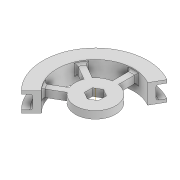
# Autodesk Inventor part: Primary_hinge_guide_pulley_fix
Saved by Autodesk Inventor 2022 (Build 260153000, 153)
## iProperties
Created: 2022-09-24
Part Number: Primary_hinge_guide_pulley_fix
Material: Generic
Document SubType Name: Modeling
Designer: dell
Density: 1 g/cm^3
Appearance: Default
Author: dell
Autodesk Inventor part; units mm, degrees
ref_plane "YZ Plane" through (0, 0, 0) normal (1, 0, 0) x (0, 1, 0)
ref_plane "XZ Plane" through (0, 0, 0) normal (0, 1, 0) x (-1, 0, 0)
ref_plane "XY Plane" through (0, 0, 0) normal (0, 0, 1) x (1, 0, 0)
sketch "Sketch1" plane through (0, 0, 0) normal (0, 1, 0) x (-1, 0, 0)
  circle A0 centre (0, 0) radius 2.05
  circle A1 centre (0, 0) radius 22
  dimension "d0" = 4.1
  dimension "d1" = 44
  constraints: 2 centre point, 2 coincident
  measures "d0" diameter of A0
  measures "d1" diameter of A1
extrude "Extrusion1" add sketch "Sketch1" along normal blind 3.7
sketch "Sketch5" plane through (0, 3.7, 0) normal (0, 1, 0) x (1, 0, 0)
  circle A0 centre (0, 0) radius 22 projected
  circle A1 centre (0, 0) radius 2.05 projected
  circle A2 centre (0, 0) radius 26
  circle A3 centre (0, 0) radius 19
  dimension "d11" = 4
  dimension "d17" = 3
  constraints: 2 centre point
  measures "d11" radial gap between concentric circles of A0 A2
  measures "d17" radial gap between concentric circles of A0 A3
extrude "Extrusion4" add sketch "Sketch5" along normal blind 1.5 contours A0 | A2
sketch "Sketch11" plane through (0, 0, 0) normal (0, -1, 0) x (1, 0, 0)
  circle A0 centre (0, 0) radius 22 projected
  circle A1 centre (0, 0) radius 2.05 projected
  circle A2 centre (0, 0) radius 19
  dimension "d38" = 3
  constraints: 1 centre point
  measures "d38" radial gap between concentric circles of A0 A2
extrude "Extrusion10" add sketch "Sketch11" along normal blind 3 contours A0
sketch "Sketch6" plane through (0, -3, 0) normal (0, -1, 0) x (1, 0, 0)
  circle A0 centre (0, 0) radius 2.05 projected
  circle A1 centre (0, 0) radius 26
  circle A2 centre (0, 0) radius 19
  constraints: 2 centre point
extrude "Extrusion5" add sketch "Sketch6" along normal blind 1.5 contours A1
sketch "Sketch7" plane through (0, 3.7, 0) normal (0, 1, 0) x (1, 0, 0)
  circle A0 centre (0, 0) radius 19
  circle A1 centre (0, 0) radius 22
  circle A2 centre (0, 0) radius 10
  line L0 (-1.5, 9.88686) -> (-1.5, 18.940697)
  circle A3 centre (0, 0) radius 19
  line L1 (1.5, 9.88686) -> (1.5, 18.940697)
  line L2 (-7.812272, 6.242468) -> (-15.653125, 10.769387)
  line L3 (-9.312272, 3.644392) -> (-17.153125, 8.17131)
  line L4 (-9.312272, -3.644392) -> (-17.153125, -8.17131)
  line L5 (-7.812272, -6.242468) -> (-15.653125, -10.769387)
  line L6 (-1.5, -9.88686) -> (-1.5, -18.940697)
  line L7 (1.5, -9.88686) -> (1.5, -18.940697)
  line L8 (7.812272, -6.242468) -> (15.653125, -10.769387)
  line L9 (9.312272, -3.644392) -> (17.153125, -8.17131)
  line L10 (9.312272, 3.644392) -> (17.153125, 8.17131)
  line L11 (7.812272, 6.242468) -> (15.653125, 10.769387)
  point P0 (1.5, 18.940697)
  point P1 (-1.5, 18.940697)
  point P2 (-9.312272, -3.644392)
  point P3 (-9.312272, 3.644392)
  point P4 (-1.5, -18.940697)
  point P5 (-1.5, -9.88686)
  point P6 (-7.812272, -6.242468)
  point P7 (-15.653125, -10.769387)
  point P8 (7.812272, -6.242468)
  point P9 (1.5, -18.940697)
  point P10 (9.312272, 3.644392)
  point P11 (7.812272, 6.242468)
  dimension "d19" = 20
  dimension "d20" = 3
  dimension "d21" = 1.5
  dimension "d26" = 360
  constraints: 24 end point, 4 point on circle, 1 centre point, 1 coincident, 1 parallel, 1 vertical, 37 other
  measures "d19" diameter of A2
  measures "d20" distance between parallel lines of L0 L1
  measures "d21" distance from line of point (0, 0) L0
extrude "Extrusion7" cut sketch "Sketch7" against normal blind 10 contours A0 L9 A2 L10 | L11 A2 L1 A0 | A0 L7 A2 L8 | L0 A2 L2 A0 | A0 L5 A2 L6 | L3 A2 L4 A0
sketch "Sketch8" plane through (0, 3.7, 0) normal (0, 1, 0) x (1, 0, 0)
  line L0 (0, -4.041452) -> (-3.5, -2.020726)
  line L1 (-3.5, -2.020726) -> (-3.5, 2.020726)
  line L2 (-3.5, 2.020726) -> (0, 4.041452)
  line L3 (0, 4.041452) -> (3.5, 2.020726)
  line L4 (3.5, 2.020726) -> (3.5, -2.020726)
  line L5 (3.5, -2.020726) -> (0, -4.041452)
  point P0 (0, 0)
  point P1 (0, 0)
  dimension "d30" = 7
  constraints: 12 end point, 1 coincident, 13 other
  measures "d30" distance between parallel lines of L4 L1
extrude "Extrusion8" cut sketch "Sketch8" against normal blind 10
fillet "Fillet1" radius 1 2 edges at (22, 3.7, 0) (-22, -3, 0)
sketch "Sketch9" plane through (0, 5.2, 0) normal (0, 1, 0) x (1, 0, 0)
  line L0 (0, 0) -> (-18.384776, -18.384776)
  circle A0 centre (0, 0) radius 26
  line L1 (0, 0) -> (13, 22.51666)
  line L2 (0, 36.4) -> (0, -36.4)
  circle A1 centre (0, 0) radius 10
  point P0 (5, 8.660254)
  point P1 (-7.071068, -7.071068)
  dimension "d34" = 150
  dimension "d35" = 45
  dimension "d41" = 20
  constraints: 4 end point, 2 point on circle, 1 centre point, 1 coincident
  measures "d34" angle of L2 L1
  measures "d35" angle of L2 L0
  measures "d41" diameter of A1
extrude "Extrusion9" cut sketch "Sketch9" against normal blind 10 contours A1 L2 A0 L0 | L1 A0 L2 A1 picked at (-2.341084, -20.43609) picked at (20.365802, -2.670251)
fillet "Fillet2" radius 1 12 edges at (-17.1531, 1.85, -8.1713) (-16.4545, 3.7, -9.5) (-15.6531, 1.85, -10.7694) (-16.4545, 0, -9.5) (-16.4545, 0, 9.5) (-15.6531, 1.85, 10.7694) (-16.4545, 3.7, 9.5) (-17.1531, 1.85, 8.1713) (1.5, 1.85, -18.9407) (0, 0, -19) (-1.5, 1.85, -18.9407) (0, 3.7, -19)
equation "\"d21\" = 0.5 * d20"
body "Solid1"
